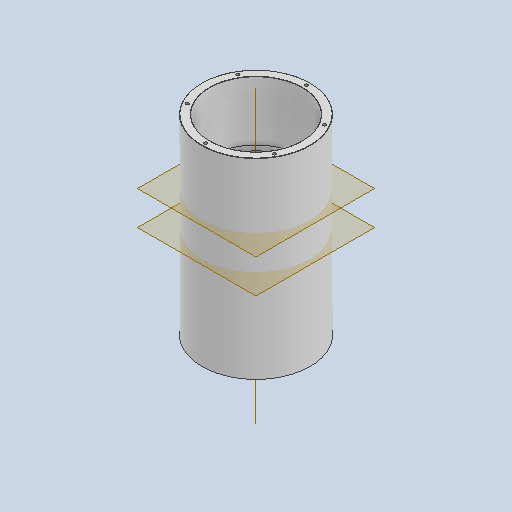
# Autodesk Inventor part: Gehäuse
Saved by Autodesk Inventor 2025 (Build 290162000, 162)
## iProperties
Created: 2022-11-23
Part Number: Gehäuse
Material: Generisch
Document SubType Name: Modeling
Designer: schil
Density: 1 g/cm^3
Appearance: Vorgabe
Author: schil
Autodesk Inventor part; units mm, degrees
ref_plane "YZ Plane" through (0, 0, 0) normal (1, 0, 0) x (0, 1, 0)
ref_plane "XZ Plane" through (0, 0, 0) normal (0, 1, 0) x (-1, 0, 0)
ref_plane "XY Plane" through (0, 0, 0) normal (0, 0, 1) x (1, 0, 0)
sketch "Skizze1" plane through (0, 0, 0) normal (1, 0, 0) x (0, 1, 0)
  line L0 (204.625, 55) -> (0, 55)
  line L1 (0, 55) -> (0, 47)
  line L2 (0, 47) -> (204.625, 47)
  line L3 (204.625, 47) -> (204.625, 55)
  line L4 (0, 47) -> (8, 47)
  line L5 (8, 47) -> (8, 0)
  line L6 (8, 0) -> (0, 0)
  line L7 (0, 0) -> (0, 47)
  line L8 (-40.925, 0) -> (245.55, 0) projected
  line L9 (0, -11) -> (0, 66) projected
  point P0 (0, 0)
  point P1 (4, 0)
  dimension "d0" = 8
  dimension "d1" = 8
  dimension "d2" = 204.625
  dimension "d3" = 47
  dimension "d4" = 0
  dimension "d5" = 0
  constraints: 16 end point, 4 parallel, 2 horizontal, 2 perpendicular, 1 midpoint
  measures "d0" distance between parallel lines of L2 L0
  measures "d1" distance between parallel lines of L7 L5
  measures "d2" distance of L1.end L2.end
  measures "d3" distance of L6.end L1.end
  measures "d4" distance between parallel lines of L9 L7
  measures "d5" distance from line of L8 point (4, 0)
revolve "Umdrehung1" add sketch "Skizze1" angle 360 about axis through (0, -10, 0) along (0, 1, 0)
sketch "Skizze2" plane through (0, 204.625, 0) normal (0, 1, 0) x (1, 0, 0)
  circle A0 centre (0, 0) radius 51 construction
  circle A1 centre (0, 0) radius 55 projected
  circle A2 centre (0, 0) radius 51 construction
  circle A3 centre (0, 0) radius 51 construction
  circle A4 centre (0, 0) radius 51 construction
  circle A5 centre (0, 0) radius 51 construction
  circle A6 centre (0, 0) radius 51 construction
  point P0 (0, -51)
  point P1 (44.1673, -25.5)
  point P2 (44.1673, 25.5)
  point P3 (0, 51)
  point P4 (-44.1673, 25.5)
  point P5 (-44.1673, -25.5)
  dimension "d16" = 4
  dimension "d19" = 360
  constraints: 8 coincident, 2 vertical alignment, 39 other
hole "Bohrung1" at (0, 204.625, 51) at (44.1673, 204.625, 25.5) at (44.1673, 204.625, -25.5) at (0, 204.625, -51) at (-44.1673, 204.625, -25.5) at (-44.1673, 204.625, 25.5) direction (0, -1, 0) diameter 3.242 depth 11.8 tip angle 118 thread size "M4x0.7" class "6H" standard "ISO Metric profile"
chamfer "Fase1" distance 0.25 angle 45 1 edges at (0, 204.625, -47)
chamfer "Fase2" distance 0.25 angle 45 1 edges at (0, 204.625, -55)
chamfer "Fase3" distance 0.25 angle 45 1 edges at (0, 0, -55)
sketch "Skizze3" plane through (0, 0, 0) normal (0, -1, 0) x (1, 0, 0)
  circle A0 centre (0, 0) radius 60.1977
  constraints: 1 centre point, 1 coincident
extrude "Extrusion1" cut sketch "Skizze3" against normal blind 10
ref_plane "Arbeitsebene1" through (0, 104.8125, 0) normal (0, 1, 0) x (1, 0, 0)
mirror "Spiegeln1" about plane through (0, 104.8125, 0) normal (0, 1, 0) of "Bohrung1"
ref_plane "Arbeitsebene3" through (0, 139.125, 0) normal (0, 1, 0) x (1, 0, 0)
sketch "Skizze4" plane through (0, 139.125, 0) normal (0, 1, 0) x (1, 0, 0)
  circle A0 centre (0, 0) radius 47 projected
  circle A1 centre (0, 0) radius 47 projected
  circle A2 centre (0, 0) radius 47
  circle A3 centre (0, 0) radius 47 projected
  circle A4 centre (0, 0) radius 40
  dimension "d33" = 7
  constraints: 2 centre point, 2 coincident, 1 concentric
  measures "d33" radial gap between concentric circles of A4 A0
extrude "Extrusion2" add sketch "Skizze4" along normal blind 5
sketch "Skizze5" plane through (0, 204.625, 0) normal (0, 1, 0) x (1, 0, 0)
  point P0 (-44.1673, -25.5)
hole "Bohrung2" at (-44.1673, 204.625, 25.5) direction (0, -1, 0) diameter 3.242 depth 8 tip angle 120 thread size "M4x0.7" class "6H" standard "ISO Metric profile"
